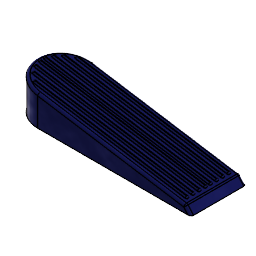
Door Stop (Autodesk Fusion 360 design; units mm, degrees)
part number: 2026-02-14-14-57-29-341
Autodesk Fusion 360 part; units mm, degrees
box "BoxPrimitive2" add length 45.72 width 127 height 5.08 placed x (0, 1, 0) y (-1, 0, 0) z (0, 0, 1) at (127, 0, 0)
cylinder "CylinderPrimitive1" add diameter 45.72 height -5.08 placed x (1, 0, 0) y (0, 1, 0) z (0, 0, 1) at (0, 22.86, 5.08)
draft "Draft1" angle 9 neutral plane through (127, 0, 0) pull (1, 0, 0) 1 faces at (84.6667, 15.24, 5.08)
chamfer "Chamfer1" distance 5.08 angle 45 1 edges at (127, 22.86, 5.08)
shell "Shell1" thickness 2.54 removed faces 2 at (127, 30.48, 0.0003) at (84.6667, 15.24, 0)
fillet "Fillet1" radius 2.032 6 edges at (60.9913, 45.72, 15.5348) (-22.86, 22.86, 28.8155) (60.9913, 0, 15.5348) (121.9825, 22.86, 5.8747) (124.4913, 0, 2.9373) (124.4913, 45.72, 2.9373)
sketch "Sketch4" plane through (3.8928, 0, 24.5783) normal (0.156434, 0, 0.987688) x (0, 1, 0)
  line L0 (43.688, -118.8121) -> (43.688, 3.6195)
  ellipse E0 centre (22.86, 3.6195) end of major axis (22.86, 24.7071) minor radius 20.828 (43.688, 3.6195) -> (2.032, 3.6195) ccw
  line L1 (2.032, 3.6195) -> (2.032, -118.8121)
  line L2 (2.032, -118.8121) -> (43.688, -118.8121)
  line L3 (6.772, -115.2546) -> (6.772, 33.3027)
  line L4 (6.772, 33.3027) -> (4.232, 33.3027)
  line L5 (4.232, 33.3027) -> (4.232, -115.2546)
  arc A0 (4.232, -115.2546) -> (6.772, -115.2546) centre (5.502, -115.2546) ccw
  line L6 (9.312, 33.3027) -> (9.312, -115.2546)
  line L7 (11.852, -115.2546) -> (11.852, 33.3027)
  line L8 (11.852, 33.3027) -> (9.312, 33.3027)
  arc A1 (9.312, -115.2546) -> (11.852, -115.2546) centre (10.582, -115.2546) ccw
  line L9 (14.392, 33.3027) -> (14.392, -115.2546)
  line L10 (16.932, -115.2546) -> (16.932, 33.3027)
  line L11 (16.932, 33.3027) -> (14.392, 33.3027)
  arc A2 (14.392, -115.2546) -> (16.932, -115.2546) centre (15.662, -115.2546) ccw
  line L12 (19.472, 33.3027) -> (19.472, -115.2546)
  line L13 (22.012, -115.2546) -> (22.012, 33.3027)
  line L14 (22.012, 33.3027) -> (19.472, 33.3027)
  arc A3 (19.472, -115.2546) -> (22.012, -115.2546) centre (20.742, -115.2546) ccw
  circle A4 centre (5.502, 11.7445) radius 1.27
  circle A5 centre (10.582, 17.5911) radius 1.27
  circle A6 centre (15.662, 21.1183) radius 1.27
  circle A7 centre (20.742, 22.4362) radius 1.27
  line L15 (22.86, 0) -> (22.86, -133.0564) construction
  line L16 (22.86, 0) -> (22.86, -133.0564) construction
  arc A8 (33.868, -115.2546) -> (36.408, -115.2546) centre (35.138, -115.2546) ccw
  line L17 (33.868, -115.2546) -> (33.868, 33.3027)
  line L18 (43.688, 3.6195) -> (43.688, -118.8121)
  arc A9 (38.948, -115.2546) -> (41.488, -115.2546) centre (40.218, -115.2546) ccw
  line L19 (33.868, 33.3027) -> (36.408, 33.3027)
  line L20 (41.488, 33.3027) -> (41.488, -115.2546)
  circle A10 centre (35.138, 17.5911) radius 1.27
  circle A11 centre (40.218, 11.7445) radius 1.27
  line L21 (23.708, -115.2546) -> (23.708, 33.3027)
  arc A12 (28.788, -115.2546) -> (31.328, -115.2546) centre (30.058, -115.2546) ccw
  circle A13 centre (24.978, 22.4362) radius 1.27
  line L22 (28.788, -115.2546) -> (28.788, 33.3027)
  line L23 (23.708, 33.3027) -> (26.248, 33.3027)
  line L24 (26.248, 33.3027) -> (26.248, -115.2546)
  line L25 (28.788, 33.3027) -> (31.328, 33.3027)
  line L26 (31.328, 33.3027) -> (31.328, -115.2546)
  line L27 (36.408, 33.3027) -> (36.408, -115.2546)
  circle A14 centre (30.058, 21.1183) radius 1.27
  line L28 (38.948, 33.3027) -> (41.488, 33.3027)
  arc A15 (23.708, -115.2546) -> (26.248, -115.2546) centre (24.978, -115.2546) ccw
  line L29 (38.948, -115.2546) -> (38.948, 33.3027)
  point P0 (45.72, 0)
  point P1 (22.86, 3.6195)
  dimension "d23" = 2.54
  dimension "d26" = 15.24
  dimension "d27" = 0
  constraint vertical L3
  constraint horizontal L4
  constraint vertical L5
  constraint tangent L5 A4
  constraint tangent L3 A4
  constraint tangent L6 A5
  constraint tangent L7 A5
  constraint tangent L9 A6
  constraint tangent L10 A6
  constraint tangent L12 A7
  constraint tangent L13 A7
  constraint perpendicular L2 L15
  constraint symmetric origin L15 P0
  constraint symmetric L1.start L15 L0.end
  constraint symmetric P1 L15 E0.centre
  constraint symmetric L1.end L15 L0.start
  constraint symmetric L5.end L15 A9.end
  constraint symmetric L3.start L15 A9.start
  constraint symmetric L3.end L15 L28.start
  constraint symmetric L4.end L15 L20.start
  constraint symmetric A0 L15 A9
  constraint symmetric L6.start L15 L19.end
  constraint symmetric L6.end L15 A8.end
  constraint symmetric L7.start L15 A8.start
  constraint symmetric L7.end L15 L17.end
  constraint symmetric A1 L15 A8
  constraint symmetric L9.start L15 L25.end
  constraint symmetric L9.end L15 A12.end
  constraint symmetric L10.start L15 A12.start
  constraint symmetric L10.end L15 L22.end
  constraint symmetric A2 L15 A12
  constraint symmetric L12.start L15 L23.end
  constraint symmetric L12.end L15 L24.end
  constraint symmetric L13.start L15 L21.start
  constraint symmetric L13.end L15 L21.end
  constraint symmetric A3 L15 A15
  constraint symmetric A4 L15 A11
  constraint symmetric A5 L15 A10
  constraint symmetric A6 L15 A14
  constraint symmetric A7 L15 A13
  constraint symmetric L16.start L15 L15.start
  constraint symmetric L16.end L15 L15.end
  measures "d23" distance of L5.end L3.start
sketch "Sketch5" plane through (3.8928, 0, 24.5783) normal (0.156434, 0, 0.987688) x (0, 1, 0)
extrude "Extrude1" add sketch "Sketch4" along normal blind 1.27 contours A11 | A9 L20 A11 L29 | L3 L5 A0 A4 | A4 | A10 | A8 L17 A10 L27 | L6 L7 A1 A5 | A5 | A14 | A12 L22 L26 A14 | L9 L10 A2 A6 | A6 | A13 | L21 A13 L24 A15 | L12 L13 A3 A7 | A7
fillet "Fillet2" radius 1.016 32 edges at (55.2094, 6.772, 17.7364) (-8.7628, 5.502, 27.8685) (55.2094, 4.232, 17.7364) (119.1815, 5.502, 7.6042) (52.322, 11.852, 18.1937) (-14.5374, 10.582, 28.7832) (52.322, 9.312, 18.1937) (119.1815, 10.582, 7.6042) (50.5802, 16.932, 18.4695) (-18.0212, 15.662, 29.3349) (50.5802, 14.392, 18.4695) (119.1815, 15.662, 7.6042) (49.9293, 22.012, 18.5726) (-19.3228, 20.742, 29.5411) (49.9293, 19.472, 18.5726) (119.1815, 20.742, 7.6042) (49.9293, 23.708, 18.5726) (119.1815, 24.978, 7.6042) (49.9293, 26.248, 18.5726) (-19.3228, 24.978, 29.5411) (50.5802, 31.328, 18.4695) (-18.0212, 30.058, 29.3349) (50.5802, 28.788, 18.4695) (119.1815, 30.058, 7.6042) (52.322, 36.408, 18.1937) (-14.5374, 35.138, 28.7832) (52.322, 33.868, 18.1937) (119.1815, 35.138, 7.6042) (55.2094, 38.948, 17.7364) (119.1815, 40.218, 7.6042) (55.2094, 41.488, 17.7364) (-8.7628, 40.218, 27.8685)
